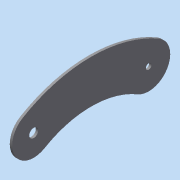
# Autodesk Inventor part: Cannon
Saved by Autodesk Inventor 2015 (Build 190159000, 159)
## iProperties
Created: 2014-09-22
Part Number: Cannon
Material: Generic
Document SubType Name: Modeling
Designer: Ashwin
Density: 1 g/cm^3
Appearance: Default
Author: Ashwin
Autodesk Inventor part; units mm, degrees
ref_plane "YZ Plane" through (0, 0, 0) normal (1, 0, 0) x (0, 1, 0)
ref_plane "XZ Plane" through (0, 0, 0) normal (0, 1, 0) x (-1, 0, 0)
ref_plane "XY Plane" through (0, 0, 0) normal (0, 0, 1) x (1, 0, 0)
sketch "Sketch1" plane through (0, 0, 0) normal (1, 0, 0) x (0, 1, 0)
  line L0 (0, 0) -> (0.0002, -101.6)
  arc A0 (0.0002, -101.6) -> (0, 0) centre (-86.1502, -50.8002) ccw construction
  arc A1 (16.4098, -111.2761) -> (16.4096, 9.6762) centre (-86.1502, -50.8002) ccw
  arc A2 (-16.4094, -91.9239) -> (-16.4096, -9.6762) centre (-86.1502, -50.8002) ccw
  arc A3 (-16.4094, -91.9239) -> (16.4098, -111.2761) centre (0.0002, -101.6) ccw
  arc A4 (16.4096, 9.6762) -> (-16.4096, -9.6762) centre (0, 0) ccw
  circle A5 centre (0, 0) radius 3.9688
  circle A6 centre (0.0002, -101.6) radius 3.9688
  dimension "d9" = 101.6
  dimension "d10" = 38.1
  dimension "d13" = 7.9375
  dimension "d14" = 7.9375
  constraints: 10 point on circle, 7 centre point, 4 tangent, 2 coincident, 2 end point
  measures "d9" distance of L0.start L0.end
  measures "d10" diameter of A3
  measures "d13" diameter of A5
  measures "d14" diameter of A6
extrude "Extrusion1" add sketch "Sketch1" along normal blind 2.1082 contours A6 | A5 | A3 A2 A4 A1
sketch "Sketch3" plane through (2.1082, 0, 0) normal (1, 0, 0) x (0, 0, -1)
  circle A0 centre (0, 0) radius 3.9688
  arc A1 (91.9239, -16.4094) -> (111.2761, 16.4098) centre (101.6, 0.0002) ccw projected
  circle A2 centre (101.6, 0.0002) radius 2.5
  dimension "d19" = 7.9375
  dimension "d20" = 5
  constraints: 2 centre point, 2 coincident
  measures "d19" diameter of A0
  measures "d20" diameter of A2
extrude "Extrusion3" cut sketch "Sketch3" against normal through all
equation "\"d21\" = d20"
body "Solid1"
